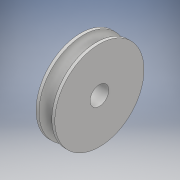
# Autodesk Inventor part: Spacer
Saved by Autodesk Inventor 2017 (Build 210142000, 142)
## iProperties
Created: 2019-06-22
Part Number: Spacer
Material: Generic
Document SubType Name: Modeling
Designer: Ole Simmering
Density: 1 g/cm^3
Appearance: Default
Author: Ole Simmering
Autodesk Inventor part; units mm, degrees
ref_plane "YZ Plane" through (0, 0, 0) normal (1, 0, 0) x (0, 1, 0)
ref_plane "XZ Plane" through (0, 0, 0) normal (0, 1, 0) x (-1, 0, 0)
ref_plane "XY Plane" through (0, 0, 0) normal (0, 0, 1) x (1, 0, 0)
sketch "Sketch1" plane through (0, 0, 0) normal (0, 0, 1) x (1, 0, 0)
  line L0 (-17.4415, 0) -> (0, 0) construction
  line L1 (0, 9.5) -> (-0.6349, 9.5)
  arc A0 (-3.3651, 9.5) -> (-0.6349, 9.5) centre (-2, 9.5) ccw
  line L2 (-3.3651, 9.5) -> (-4, 9.5)
  line L3 (-2, 9.5) -> (-2, 2.9223) construction
  line L4 (-4, 9.5) -> (-4, 2)
  line L5 (-4, 2) -> (0, 2)
  line L6 (0, 2) -> (0, 9.5)
  dimension "d1" = 4
  dimension "d2" = 19
  dimension "d3" = 1.3651
  dimension "d4" = 4
  constraints: 14 end point, 4 point on line, 2 horizontal, 2 perpendicular, 2 point on circle, 2 vertical, 1 centre point, 2 other
  measures "d1" diameter of L5 L0
  measures "d2" diameter of L2 L0
  measures "d3" radius of A0
  measures "d4" distance of L4.end L5.end
revolve "Revolution1" add sketch "Sketch1" angle 360 about axis through (-17.4415, 0, 0) along (1, 0, 0)
body "Solid1"
